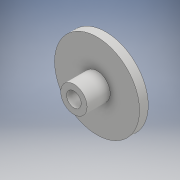
# Autodesk Inventor part: inner_wheel
Saved by Autodesk Inventor 2017 (Build 210142000, 142)
## iProperties
Created: 2017-04-01
Part Number: inner_wheel
Material: Generic
Document SubType Name: Modeling
Designer: Nick
Density: 1 g/cm^3
Appearance: Default
Author: Nick
Autodesk Inventor part; units mm, degrees
ref_plane "YZ Plane" through (0, 0, 0) normal (1, 0, 0) x (0, 1, 0)
ref_plane "XZ Plane" through (0, 0, 0) normal (0, 1, 0) x (-1, 0, 0)
ref_plane "XY Plane" through (0, 0, 0) normal (0, 0, 1) x (1, 0, 0)
sketch "Sketch1" plane through (0, 0, 0) normal (0, 1, 0) x (-1, 0, 0)
  circle A0 centre (0, 0) radius 14.5
  dimension "d0" = 29
  constraints: 1 centre point, 1 coincident
  measures "d0" diameter of A0
extrude "Extrusion1" add sketch "Sketch1" along normal blind 3
sketch "Sketch2" plane through (0, 3, 0) normal (0, 1, 0) x (1, 0, 0)
  circle A0 centre (0, 0) radius 13.5
  dimension "d3" = 27
  constraints: 1 centre point, 1 coincident
  measures "d3" diameter of A0
extrude "Extrusion2" cut sketch "Sketch2" against normal blind 0.5
sketch "Sketch3" plane through (0, 2.5, 0) normal (0, 1, 0) x (1, 0, 0)
  circle A0 centre (0, 0) radius 11
  circle A1 centre (0, 0) radius 5
  line L0 (-6.5333, 7.5044) -> (-3.8846, 4.462) construction
  line L1 (3.0432, 5.0733) -> (5.1182, 8.5325) construction
  arc A2 (4.6868, 9.9516) -> (-6.3569, 8.9771) centre (0, 0) ccw
  arc A3 (1.8214, 4.6564) -> (-2.6087, 4.2656) centre (0, 0) ccw
  line L2 (-7.2228, 8.2965) -> (-3.2831, 3.7711)
  line L3 (5.6584, 9.433) -> (2.572, 4.2877)
  arc A4 (-6.3569, 8.9771) -> (-6.5333, 7.5044) centre (-5.779, 8.161) ccw
  arc A5 (-3.8846, 4.462) -> (-2.6087, 4.2656) centre (-3.1304, 5.1187) ccw
  arc A6 (1.8214, 4.6564) -> (3.0432, 5.0733) centre (2.1857, 5.5877) ccw
  arc A7 (5.1182, 8.5325) -> (4.6868, 9.9516) centre (4.2607, 9.0469) ccw
  arc A8 (3.0991, 9.499) -> (-4.7146, 8.8096) centre (0.0131, -0.1481) ccw
  arc A9 (1.4786, 5.8357) -> (-2.4777, 5.4866) centre (-0.0344, 0.3898) ccw
  line L4 (-5.0021, 7.2686) -> (-3.6641, 5.7318)
  line L5 (3.652, 8.0321) -> (2.6039, 6.2848)
  arc A10 (-4.7146, 8.8096) -> (-5.0021, 7.2686) centre (-4.2478, 7.9252) ccw
  arc A11 (-3.6641, 5.7318) -> (-2.4777, 5.4866) centre (-2.9099, 6.3884) ccw
  arc A12 (1.4786, 5.8357) -> (2.6039, 6.2848) centre (1.7463, 6.7992) ccw
  arc A13 (3.652, 8.0321) -> (3.0991, 9.499) centre (2.7944, 8.5466) ccw
  arc A14 (9.9918, -0.0121) -> (6.9215, 7.2061) centre (-0.1369, -0.0582) ccw
  arc A15 (6.9215, 7.2061) -> (5.3671, 7.0033) centre (6.2246, 6.4889) ccw
  line L6 (5.3671, 7.0033) -> (4.319, 5.256)
  arc A16 (4.319, 5.256) -> (4.4525, 4.0519) centre (5.1765, 4.7416) ccw
  arc A17 (6.007, 0.3971) -> (4.4525, 4.0519) centre (0.3601, 0.1532) ccw
  arc A18 (6.007, 0.3971) -> (6.7819, -0.5343) centre (7.0061, 0.4402) ccw
  line L7 (8.7676, -0.9912) -> (6.7819, -0.5343)
  arc A19 (8.7676, -0.9912) -> (9.9918, -0.0121) centre (8.9918, -0.0166) ccw
  arc A20 (3.0761, -9.5065) -> (8.9923, -4.3559) centre (-0.0977, 0.1122) ccw
  arc A21 (8.9923, -4.3559) -> (8.3191, -2.9403) centre (8.0949, -3.9148) ccw
  line L8 (8.3191, -2.9403) -> (6.3334, -2.4834)
  arc A22 (6.3334, -2.4834) -> (5.2294, -2.9825) centre (6.1092, -3.4579) ccw
  arc A23 (2.2339, -5.5903) -> (5.2294, -2.9825) centre (0.2569, -0.2951) ccw
  arc A24 (2.2339, -5.5903) -> (1.5876, -6.615) centre (2.5837, -6.5271) ccw
  line L9 (1.7667, -8.6447) -> (1.5876, -6.615)
  arc A25 (1.7667, -8.6447) -> (3.0761, -9.5065) centre (2.7628, -8.5568) ccw
  arc A26 (-8.0906, -5.8632) -> (-1.3639, -9.8982) centre (0.0765, 0.1275) ccw
  arc A27 (-1.3639, -9.8982) -> (-0.2256, -8.8205) centre (-1.2217, -8.9084) ccw
  line L10 (-0.2256, -8.8205) -> (-0.4047, -6.7908)
  arc A28 (-0.4047, -6.7908) -> (-1.2205, -5.8951) centre (-1.4008, -6.8787) ccw
  arc A29 (-4.6264, -3.8521) -> (-1.2205, -5.8951) centre (-0.2013, -0.3355) ccw
  arc A30 (-4.6264, -3.8521) -> (-5.8007, -3.554) centre (-5.4093, -4.4742) ccw
  line L11 (-7.6757, -4.3516) -> (-5.8007, -3.554)
  arc A31 (-7.6757, -4.3516) -> (-8.0906, -5.8632) centre (-7.2843, -5.2718) ccw
  arc A32 (-8.0764, 5.8828) -> (-9.8353, -1.7615) centre (0.1449, -0.0333) ccw
  arc A33 (-9.8353, -1.7615) -> (-8.4585, -2.5111) centre (-8.8499, -1.5909) ccw
  line L12 (-8.4585, -2.5111) -> (-6.5835, -1.7136)
  arc A34 (-6.5835, -1.7136) -> (-5.9837, -0.6609) centre (-6.9749, -0.7934) ccw
  arc A35 (-5.0932, 3.2096) -> (-5.9837, -0.6609) centre (-0.3813, 0.0877) ccw
  arc A36 (-5.0932, 3.2096) -> (-5.1726, 4.4185) centre (-5.9268, 3.7619) ccw
  line L13 (-6.5105, 5.9553) -> (-5.1726, 4.4185)
  arc A37 (-6.5105, 5.9553) -> (-8.0764, 5.8828) centre (-7.2647, 5.2987) ccw
  point P0 (-10.1224, -4.3055)
  point P1 (0.9668, -10.9574)
  point P2 (10.7199, -2.4665)
  point P3 (-5.779, 8.161)
  point P4 (-3.1304, 5.1187)
  point P5 (2.1857, 5.5877)
  point P6 (3.9008, 4.5589)
  point P7 (5.9897, -0.352)
  point P8 (5.5412, -2.3011)
  point P9 (1.5161, -5.8053)
  point P10 (-0.4761, -5.9811)
  point P11 (-5.0527, -3.2358)
  point P12 (-5.8355, -1.3954)
  point P13 (-4.6388, 3.8054)
  dimension "d6" = 22
  dimension "d7" = 10
  dimension "d10" = 360
  dimension "d12" = 1
  dimension "d13" = 1
  dimension "d14" = 1
  dimension "d17" = 360
  constraints: 92 point on circle, 37 centre point, 28 end point, 18 point on line, 16 tangent, 6 coincident, 5 equal radius, 2 collinear, 1 concentric, 136 other
  measures "d7" diameter of A1
  measures "d12" radius of A4
  measures "d13" radius of A5
  measures "d14" radius of A10
extrude "Extrusion3" cut sketch "Sketch3" against normal blind 0.4 contours A13 L5 A12 A9 A11 L4 A10 A8 | A19 L7 A18 A17 A16 L6 A15 A14 | A25 L9 A24 A23 A22 L8 A21 A20 | A31 L11 A30 A29 A28 L10 A27 A26 | A37 L13 A36 A35 A34 L12 A33 A32
sketch "Sketch4" plane through (0, 2.5, 0) normal (0, 1, 0) x (1, 0, 0)
  circle A0 centre (0, 0) radius 4
  dimension "d21" = 8
  constraints: 1 centre point, 1 coincident
  measures "d21" diameter of A0
extrude "Extrusion4" add sketch "Sketch4" along normal blind 0.6
sketch "Sketch5" plane through (0, 3.1, 0) normal (0, 1, 0) x (1, 0, 0)
  circle A0 centre (0, 0) radius 2.5
  dimension "d24" = 5
  constraints: 1 centre point, 1 coincident
  measures "d24" diameter of A0
extrude "Extrusion5" cut sketch "Sketch5" against normal blind 14.15
sketch "Sketch6" plane through (0, 0, 0) normal (0, -1, 0) x (1, 0, 0)
  circle A0 centre (0, 0) radius 2.5 projected
  circle A1 centre (0, 0) radius 4.5
  dimension "d27" = 9
  constraints: 1 centre point, 1 coincident
  measures "d27" diameter of A1
extrude "Extrusion6" add sketch "Sketch6" along normal blind 7.9
body "Solid1"
